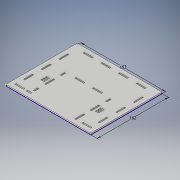
# Autodesk Inventor part: base_v2
Saved by Autodesk Inventor 2017.2 (Build 212233000, 233)
## iProperties
Created: 2017-06-08
Part Number: base_v2
Material: Generic
Document SubType Name: Modeling
Designer: SandeepSH
Density: 1 g/cm^3
Appearance: Default
Author: SandeepSH
Autodesk Inventor part; units mm, degrees
ref_plane "YZ Plane" through (0, 0, 0) normal (1, 0, 0) x (0, 1, 0)
ref_plane "XZ Plane" through (0, 0, 0) normal (0, 1, 0) x (-1, 0, 0)
ref_plane "XY Plane" through (0, 0, 0) normal (0, 0, 1) x (1, 0, 0)
sketch "Sketch1" plane through (0, 0, 0) normal (0, 1, 0) x (-1, 0, 0)
  line L0 (0, 0) -> (-192, 0)
  line L1 (-192, 0) -> (-192, -162)
  line L2 (-192, -162) -> (0, -162)
  line L3 (0, -162) -> (0, 0)
  dimension "d0" = 192
  dimension "d1" = 162
  constraints: 8 end point, 2 parallel, 1 horizontal, 1 perpendicular
  measures "d0" distance of L2.end L1.end
  measures "d1" distance of L1.end L0.end
extrude "Extrusion1" add sketch "Sketch1" along normal blind 3
fillet "Fillet1" radius 2 4 edges at (0, 1.5, 0) (192, 1.5, 0) (0, 1.5, -162) (192, 1.5, -162) curvature continuous yes
sketch "Sketch2" plane through (0, 3, 0) normal (0, 1, 0) x (1, 0, 0)
  point P0 (0, 0)
sketch "Sketch3" plane through (0, 3, 0) normal (0, 1, 0) x (1, 0, 0)
  line L0 (26, 152) -> (46, 152)
  line L1 (46, 152) -> (46, 149)
  line L2 (46, 149) -> (26, 149)
  line L3 (26, 149) -> (26, 152)
  line L4 (190, 162) -> (2, 162) projected
  line L5 (0, 160) -> (0, 2) projected
  line L6 (66, 152) -> (86, 152)
  line L7 (86, 152) -> (86, 149)
  line L8 (86, 149) -> (66, 149)
  line L9 (66, 149) -> (66, 152)
  line L10 (106, 152) -> (126, 152)
  line L11 (126, 152) -> (126, 149)
  line L12 (126, 149) -> (106, 149)
  line L13 (106, 149) -> (106, 152)
  line L14 (146, 149) -> (166, 149)
  line L15 (166, 149) -> (166, 152)
  line L16 (166, 152) -> (146, 152)
  line L17 (146, 152) -> (146, 149)
  point P0 (0, 0)
  dimension "d5" = 20
  dimension "d6" = 3
  dimension "d7" = 10
  dimension "d8" = 26
  dimension "d9" = 20
  dimension "d10" = 3
  dimension "d11" = 20
  dimension "d12" = 20
  dimension "d13" = 20
  dimension "d14" = 3
  dimension "d15" = 20
  dimension "d16" = 20
  dimension "d20" = 3
  constraints: 32 end point, 8 parallel, 4 horizontal, 4 perpendicular, 3 collinear
  measures "d5" distance of L1.end L2.end
  measures "d6" distance of L0.end L1.end
  measures "d7" distance between parallel lines of L4 L0
  measures "d8" distance between parallel lines of L3 L5
  measures "d9" distance of L7.end L8.end
  measures "d10" distance between parallel lines of L6 L8
  measures "d11" distance between parallel lines of L1 L9
  measures "d12" distance of L11.end L12.end
  measures "d13" distance between parallel lines of L7 L13
  measures "d14" distance between parallel lines of L10 L12
  measures "d15" distance of L16.end L15.end
  measures "d16" distance between parallel lines of L17 L11
  measures "d20" distance between parallel lines of L14 L16
sketch "Sketch4" plane through (0, 3, 0) normal (0, 1, 0) x (1, 0, 0)
  line L0 (10, 30) -> (13, 30)
  line L1 (13, 30) -> (13, 50)
  line L2 (13, 50) -> (10, 50)
  line L3 (10, 50) -> (10, 30)
  line L4 (2, 0) -> (190, 0) projected
  line L5 (10, 70) -> (13, 70)
  line L6 (13, 70) -> (13, 90)
  line L7 (13, 90) -> (10, 90)
  line L8 (10, 90) -> (10, 70)
  line L9 (10, 110) -> (13, 110)
  line L10 (13, 110) -> (13, 130)
  line L11 (13, 130) -> (10, 130)
  line L12 (10, 130) -> (10, 110)
  line L13 (0, 160) -> (0, 2) projected
  line L14 (96, 70) -> (96, 162)
  line L15 (190, 162) -> (2, 162) projected
  line L16 (182, 30) -> (179, 30)
  line L17 (179, 30) -> (179, 50)
  line L18 (179, 50) -> (182, 50)
  line L19 (182, 50) -> (182, 30)
  line L20 (182, 70) -> (179, 70)
  line L21 (179, 70) -> (179, 90)
  line L22 (179, 90) -> (182, 90)
  line L23 (182, 90) -> (182, 70)
  line L24 (182, 110) -> (179, 110)
  line L25 (179, 110) -> (179, 130)
  line L26 (179, 130) -> (182, 130)
  line L27 (182, 130) -> (182, 110)
  line L28 (192, 2) -> (192, 160) projected
  point P0 (0, 0)
  dimension "d23" = 3
  dimension "d24" = 20
  dimension "d25" = 30
  dimension "d26" = 3
  dimension "d27" = 20
  dimension "d28" = 20
  dimension "d29" = 20
  dimension "d30" = 20
  dimension "d31" = 96
  dimension "d72" = 10
  dimension "d73" = 3
  dimension "d85" = 192
  constraints: 50 end point, 12 symmetric about line, 6 parallel, 3 horizontal, 3 perpendicular, 2 collinear, 1 midpoint
  measures "d23" distance of L2.end L1.end
  measures "d24" distance of L1.end L0.end
  measures "d25" distance between parallel lines of L4 L0
  measures "d26" distance of L7.end L6.end
  measures "d27" distance of L6.end L5.end
  measures "d28" distance between parallel lines of L5 L2
  measures "d29" distance of L10.end L9.end
  measures "d30" distance between parallel lines of L9 L7
  measures "d31" distance from line of L13 L14.start
  measures "d72" distance between parallel lines of L13 L8
  measures "d73" distance between parallel lines of L12 L10
  measures "d85" distance between parallel lines of L28 L13
extrude "Extrusion3" cut sketch "Sketch4" against normal through all
sketch "Sketch5" plane through (0, 3, 0) normal (0, 1, 0) x (1, 0, 0)
  line L0 (146, 30) -> (149, 30)
  line L1 (149, 30) -> (149, 10)
  line L2 (149, 10) -> (146, 10)
  line L3 (146, 10) -> (146, 30)
  line L4 (179, 30) -> (179, 50) projected
  line L5 (2, 0) -> (190, 0) projected
  line L6 (146, 45) -> (149, 45)
  line L7 (149, 45) -> (149, 65)
  line L8 (149, 65) -> (146, 65)
  line L9 (146, 65) -> (146, 45)
  line L10 (146, 90) -> (149, 90)
  line L11 (149, 90) -> (149, 80)
  line L12 (149, 80) -> (146, 80)
  line L13 (146, 80) -> (146, 90)
  line L14 (96, 70) -> (96, 17.3538)
  line L15 (46, 45) -> (43, 45)
  line L16 (43, 45) -> (43, 65)
  line L17 (43, 65) -> (46, 65)
  line L18 (46, 65) -> (46, 45)
  line L19 (46, 90) -> (43, 90)
  line L20 (43, 90) -> (43, 80)
  line L21 (43, 80) -> (46, 80)
  line L22 (46, 80) -> (46, 90)
  line L23 (43, 19) -> (46, 19)
  line L24 (46, 19) -> (46, 29)
  line L25 (46, 29) -> (43, 29)
  line L26 (43, 29) -> (43, 19)
  point P0 (0, 0)
  dimension "d34" = 3
  dimension "d35" = 20
  dimension "d36" = 30
  dimension "d37" = 10
  dimension "d38" = 20
  dimension "d39" = 15
  dimension "d40" = 3
  dimension "d41" = 10
  dimension "d42" = 15
  dimension "d43" = 50
  dimension "d57" = 3
  dimension "d58" = 10
  dimension "d59" = 19
  constraints: 50 end point, 8 parallel, 8 symmetric about line, 4 collinear, 4 horizontal, 4 perpendicular, 1 vertical
  measures "d34" distance of L1.end L2.end
  measures "d35" distance of L0.end L1.end
  measures "d36" distance between parallel lines of L4 L1
  measures "d37" distance between parallel lines of L5 L2
  measures "d38" distance of L7.end L6.end
  measures "d39" distance between parallel lines of L0 L6
  measures "d40" distance of L11.end L12.end
  measures "d41" distance of L10.end L11.end
  measures "d42" distance between parallel lines of L8 L12
  measures "d43" distance between parallel lines of L9 L14
  measures "d57" distance of L25.end L24.end
  measures "d58" distance of L24.end L23.end
  measures "d59" distance between parallel lines of L5 L23
extrude "Extrusion4" cut sketch "Sketch5" against normal through all
sketch "Sketch6" plane through (0, 3, 0) normal (0, 1, 0) x (1, 0, 0)
  line L0 (182, 10) -> (162, 10)
  line L1 (162, 10) -> (162, 13)
  line L2 (162, 13) -> (182, 13)
  line L3 (182, 13) -> (182, 10)
  line L4 (2, 0) -> (190, 0) projected
  line L5 (192, 2) -> (192, 160) projected
  line L6 (10, 10) -> (30, 10)
  line L7 (30, 10) -> (30, 13)
  line L8 (30, 13) -> (10, 13)
  line L9 (10, 13) -> (10, 10)
  line L10 (0, 160) -> (0, 2) projected
  line L11 (36, 10) -> (46, 10)
  line L12 (46, 10) -> (46, 13)
  line L13 (46, 13) -> (36, 13)
  line L14 (36, 13) -> (36, 10)
  line L15 (46, 29) -> (46, 19) projected
  point P0 (0, 0)
  dimension "d46" = 20
  dimension "d47" = 3
  dimension "d48" = 10
  dimension "d49" = 10
  dimension "d50" = 20
  dimension "d51" = 3
  dimension "d52" = 10
  dimension "d53" = 10
  dimension "d60" = 10
  dimension "d61" = 3
  constraints: 24 end point, 6 parallel, 3 horizontal, 3 perpendicular, 1 collinear
  measures "d46" distance of L1.end L2.end
  measures "d47" distance of L0.end L1.end
  measures "d48" distance between parallel lines of L4 L0
  measures "d49" distance between parallel lines of L5 L3
  measures "d50" distance of L8.end L7.end
  measures "d51" distance of L7.end L6.end
  measures "d52" distance between parallel lines of L10 L9
  measures "d53" distance between parallel lines of L4 L6
  measures "d60" distance of L13.end L12.end
  measures "d61" distance of L12.end L11.end
sketch "Sketch7" plane through (0, 3, 0) normal (0, 1, 0) x (1, 0, 0)
  line L0 (66, 90) -> (86, 90)
  line L1 (86, 90) -> (86, 93)
  line L2 (86, 93) -> (66, 93)
  line L3 (66, 93) -> (66, 90)
  line L4 (43, 90) -> (46, 90) projected
  line L5 (46, 90) -> (46, 80) projected
  line L6 (106, 90) -> (126, 90)
  line L7 (126, 90) -> (126, 93)
  line L8 (126, 93) -> (106, 93)
  line L9 (106, 93) -> (106, 90)
  line L10 (146, 80) -> (146, 90) projected
  point P0 (0, 0)
  dimension "d64" = 20
  dimension "d65" = 3
  dimension "d66" = 20
  dimension "d67" = 20
  dimension "d68" = 3
  dimension "d69" = 20
  constraints: 16 end point, 4 parallel, 2 collinear, 2 horizontal, 2 perpendicular
  measures "d64" distance of L2.end L1.end
  measures "d65" distance of L1.end L0.end
  measures "d66" distance between parallel lines of L3 L5
  measures "d67" distance of L8.end L7.end
  measures "d68" distance of L7.end L6.end
  measures "d69" distance between parallel lines of L7 L10
extrude "Extrusion6" cut sketch "Sketch7" against normal through all
sketch "Sketch8" plane through (0, 3, 0) normal (0, 1, 0) x (1, 0, 0)
  line L0 (146.6767, 55) -> (192.0193, 55)
  line L1 (86, 90) -> (66, 90) projected
  line L2 (43, 65) -> (43, 45) projected
  line L3 (38, 56.5) -> (38, 53.5)
  line L4 (38, 53.5) -> (30.5, 53.5)
  line L5 (30.5, 53.5) -> (30.5, 56.5)
  line L6 (30.5, 56.5) -> (38, 56.5)
  line L7 (38, 56.5) -> (30.5, 53.5) construction
  line L8 (38, 53.5) -> (30.5, 56.5) construction
  line L9 (96, 67.642) -> (96, 32.7104)
  line L10 (146, 45) -> (146, 65) projected
  line L11 (30.5, 58.5) -> (38, 58.5)
  line L12 (38, 58.5) -> (38, 61.5)
  line L13 (38, 61.5) -> (30.5, 61.5)
  line L14 (30.5, 61.5) -> (30.5, 58.5)
  line L15 (30.5, 51.5) -> (38, 51.5)
  line L16 (38, 51.5) -> (38, 48.5)
  line L17 (38, 48.5) -> (30.5, 48.5)
  line L18 (30.5, 48.5) -> (30.5, 51.5)
  line L19 (154, 56.5) -> (154, 53.5)
  line L20 (154, 53.5) -> (161.5, 53.5)
  line L21 (161.5, 53.5) -> (161.5, 56.5)
  line L22 (161.5, 56.5) -> (154, 56.5)
  line L23 (154, 56.5) -> (161.5, 53.5) construction
  line L24 (154, 53.5) -> (161.5, 56.5) construction
  line L25 (161.5, 58.5) -> (154, 58.5)
  line L26 (154, 58.5) -> (154, 61.5)
  line L27 (154, 61.5) -> (161.5, 61.5)
  line L28 (161.5, 61.5) -> (161.5, 58.5)
  line L29 (154, 51.5) -> (154, 48.5)
  line L30 (161.5, 48.5) -> (161.5, 51.5)
  line L31 (154, 48.5) -> (161.5, 48.5)
  line L32 (161.5, 51.5) -> (154, 51.5)
  point P0 (0, 0)
  point P1 (43, 55)
  point P2 (34.25, 55)
  point P3 (157.75, 55)
  dimension "d74" = 35
  dimension "d75" = 5
  dimension "d76" = 7.5
  dimension "d77" = 50
  dimension "d78" = 3
  dimension "d79" = 1.5
  dimension "d80" = 7.5
  dimension "d81" = 3
  dimension "d82" = 2
  constraints: 60 end point, 17 symmetric about line, 5 midpoint, 4 parallel, 2 horizontal, 2 perpendicular, 2 vertical, 1 collinear
  measures "d74" distance between parallel lines of L1 L0
  measures "d75" distance between parallel lines of L2 L3
  measures "d76" distance between parallel lines of L3 L5
  measures "d77" distance between parallel lines of L10 L9
  measures "d78" distance between parallel lines of L4 L6
  measures "d79" distance between parallel lines of L4 L0
  measures "d80" distance of L13.end L12.end
  measures "d81" distance of L12.end L11.end
  measures "d82" distance between parallel lines of L11 L6
extrude "Extrusion7" cut sketch "Sketch8" against normal through all
sketch "arduino" plane through (0, 3, 0) normal (0, 1, 0) x (1, 0, 0)
  line L0 (55, 137) -> (35, 137) projected
  line L1 (35, 137) -> (5.0623, 137)
  line L2 (13, 130) -> (13, 110) projected
  line L3 (13, 118.6544) -> (13, 143.1014)
  line L4 (13, 137) -> (67, 137)
  line L5 (67, 137) -> (67, 66)
  line L6 (67, 66) -> (13, 66)
  line L7 (13, 66) -> (13, 137)
  line L8 (30.5, 71.242) -> (30.5, 18.397)
  line L9 (46, 65) -> (46, 45) projected
  line L10 (25.5, 71.242) -> (25.5, 36.8941)
  line L11 (46, 149) -> (26, 149) projected
  line L12 (13, 149) -> (84, 149)
  line L13 (84, 149) -> (84, 95)
  line L14 (84, 95) -> (13, 95)
  line L15 (13, 95) -> (13, 149)
  line L16 (13, 140) -> (16, 140)
  line L17 (16, 140) -> (16, 128)
  line L18 (16, 128) -> (13, 128)
  line L19 (13, 128) -> (13, 140)
  point P0 (0, 0)
  dimension "d86" = 54
  dimension "d87" = 71
  dimension "d88" = 15.5
  dimension "d89" = 5
  dimension "d92" = 71
  dimension "d93" = 54
  dimension "d94" = 3
  dimension "d95" = 12
  dimension "d96" = 9
  constraints: 32 end point, 6 parallel, 4 horizontal, 4 perpendicular, 4 point on line, 2 vertical, 1 collinear
  measures "d86" distance of L5.end L6.end
  measures "d87" distance of L4.end L5.end
  measures "d88" distance between parallel lines of L9 L8
  measures "d89" distance between parallel lines of L8 L10
  measures "d92" distance of L13.end L14.end
  measures "d93" distance of L12.end L13.end
  measures "d94" distance of L17.end L18.end
  measures "d95" distance of L16.end L17.end
  measures "d96" distance between parallel lines of L12 L16
extrude "Extrusion8" cut sketch "Sketch6" against normal through all
extrude "Extrusion9" cut sketch "Sketch3" against normal through all
equation "\"d9\" = d5"
equation "\"d10\" = d6"
equation "\"d11\" = d5"
equation "\"d12\" = d5"
equation "\"d13\" = d9"
equation "\"d14\" = d10"
equation "\"d15\" = d16"
equation "\"d16\" = d12"
equation "\"d20\" = d14"
equation "\"d31\" = 0.5 * d85"
equation "\"d38\" = d35"
equation "\"d66\" = d64"
equation "\"d69\" = d66"
equation "\"d76\" = d80"
body "Solid1"
